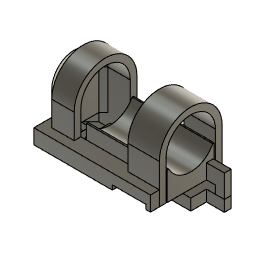
Laser Module Cover (Autodesk Fusion 360 design; units mm, degrees)
Autodesk Fusion 360 part; units mm, degrees
sketch "Sketch1" plane through (0, 0, 0) normal (1, 0, 0) x (0, 1, 0)
  line L0 (0, 0) -> (14, 0)
  line L1 (14, 0) -> (14, 8.8)
  line L2 (0, 0) -> (0, 8.8)
  arc A0 (14, 8.8) -> (0, 8.8) centre (7, 8.8) ccw
  dimension "d2" = 8.8
  dimension "d3" = 14
  constraint coincident L0.start L2.start
  constraint horizontal L0
  constraint perpendicular L0 L1
  constraint perpendicular L0 L2
  constraint tangent L1 A0
  constraint tangent L2 A0
  measures "d2" vertical distance of L0.start L2.end
  measures "d3" horizontal distance of L0.start L0.end
extrude "Extrude1" add sketch "Sketch1" along normal blind 1 makes body 1
sketch "Sketch2" plane through (1, 0, 0) normal (1, 0, 0) x (0, 1, 0)
  line L0 (0, 0) -> (14, 0)
  line L1 (14, 0) -> (14, 8.8)
  arc A0 (14, 8.8) -> (0, 8.8) centre (7, 8.8) ccw
  line L2 (0, 8.8) -> (0, 0)
  line L3 (1.5, 0) -> (1.5, 8.8)
  line L4 (12.5, 0) -> (12.5, 8.8)
  arc A1 (12.5, 8.8) -> (1.5, 8.8) centre (7, 8.8) ccw
  dimension "d6" = 1.5
  dimension "d7" = 1.5
  constraint coincident L0 L3.start
  constraint perpendicular L0 L3
  constraint coincident L0 L4.start
  constraint perpendicular L0 L4
  constraint coincident A0.centre A1.centre
  constraint tangent L3 A1
  measures "d6" distance of L2 L3
  measures "d7" distance of L1 L4
extrude "Extrude2" add sketch "Sketch2" along normal blind 6 contours L0 L1 A0 L2 L3 L4 A1 bodies 1
extrude "Extrude3" add 1 faces at (7, 13.5, 2.9333) along direction (1, 0, 0) blind 7 separate body on bodies 1 makes body 2
sketch "Sketch3" plane through (0, 0, 0) normal (0, 0, 1) x (1, 0, 0)
  line L0 (0, 0) -> (26, 0) construction
  dimension "d12" = 26
  constraint coincident L0.start origin
  measures "d12" distance of L0.start L0.end
move_body "Align1" bodies 2 to x (1, 0, 0) y (0, 1, 0) z (0, 0, 1) at (12, 0, 0)
sketch "Sketch4" plane through (0, 0, 0) normal (0, 0, -1) x (1, 0, 0)
  line L0 (0, 0) -> (0, -14)
  line L1 (0, -14) -> (7, -14)
  line L2 (7, -14) -> (7, -12.5)
  line L3 (7, -12.5) -> (1, -12.5)
  line L4 (1, -12.5) -> (1, -1.5)
  line L5 (1, -1.5) -> (7, -1.5)
  line L6 (7, -1.5) -> (7, 0)
  line L7 (7, 0) -> (0, 0)
  line L8 (0, -1.5) -> (26, -1.5)
  line L9 (26, -1.5) -> (26, 2)
  line L10 (26, 2) -> (0, 2)
  line L11 (0, 2) -> (0, -1.5)
  point P0 (26, -1.5)
  dimension "d13" = 3.5
  constraint coincident L0 L8.start
  constraint perpendicular L0 L8
  constraint perpendicular L8 L9
  constraint perpendicular L0 L10
  constraint perpendicular L8 L11
  constraint coincident P0 L8.end
  measures "d13" vertical distance of L8.start L10.end
extrude "Extrude4" add sketch "Sketch4" against normal blind 3.3 contours L6 L7 L8 L9 L10 L11 bodies 2 1
sketch "Sketch5" plane through (0, 0, 0) normal (0, 0, -1) x (1, 0, 0)
  line L0 (1, -1.5) -> (26, -1.5)
  line L1 (26, -1.5) -> (26, 0)
  line L2 (26, 0) -> (26, 2)
  line L3 (26, 2) -> (0, 2)
  line L4 (0, 2) -> (0, -14)
  line L5 (0, -14) -> (7, -14)
  line L6 (7, -14) -> (7, -12.5)
  line L7 (7, -12.5) -> (1, -12.5)
  line L8 (1, -12.5) -> (1, -1.5)
  line L9 (0, -14) -> (26, -14)
  line L10 (26, -14) -> (26, -12.5)
  line L11 (26, -12.5) -> (0, -12.5)
  line L12 (0, -12.5) -> (0, -14)
  point P0 (26, -12.5)
  constraint horizontal L9
  constraint vertical L10
  constraint horizontal L11
  constraint vertical L12
  constraint coincident P0 L10.end
  constraint coincident L4.end L5.start
extrude "Extrude5" add sketch "Sketch5" along normal blind 1.8 contours L4 L5 L6 L7 L9 L11 L12 | L6 L9 L10 L11 bodies 2
sketch "Sketch6" plane through (0, 0, 0) normal (0, 0, -1) x (1, 0, 0)
  line L0 (0, -12.5) -> (1, -12.5)
  line L1 (1, -12.5) -> (1, -1.5)
  line L2 (1, -1.5) -> (26, -1.5)
  line L3 (26, -1.5) -> (26, 0)
  line L4 (26, 0) -> (26, 2)
  line L5 (26, 2) -> (0, 2)
  line L6 (0, 2) -> (0, -12.5)
  line L7 (17.5, -1.5) -> (17.5, 2.5)
  line L8 (26, 2.5) -> (26, -1.5)
  line L9 (25, 2.5) -> (25, -1.5)
  line L10 (17.5, 2.5) -> (25, 2.5)
  line L11 (25, -1.5) -> (17.5, -1.5)
  dimension "d19" = 8.5
  dimension "d22" = 1
  constraint vertical L7
  constraint vertical L8
  constraint coincident L2 L9.end
  constraint horizontal L10
  constraint horizontal L11
  measures "d19" horizontal distance of L7.end L8.start
  measures "d22" distance of L8 L9
extrude "Extrude6" cut sketch "Sketch6" against normal blind 1 contours L5 L7 L9 L10 | L2 L5 L7 L9 L11 bodies 2
sketch "Sketch7" plane through (0, 0, -1.8) normal (0, 0, -1) x (1, 0, 0)
  line L0 (0, -12.5) -> (0, -14)
  line L1 (0, -14) -> (26, -14)
  line L2 (26, -14) -> (26, -12.5)
  line L3 (26, -12.5) -> (0, -12.5)
  line L4 (0, -14) -> (26, -14)
  line L5 (26, -14) -> (26, -7)
  line L6 (26, -7) -> (0, -7)
  line L7 (0, -7) -> (0, -14)
  line L8 (26, -14) -> (26, 0)
  dimension "d23" = 7
  constraint horizontal L4
  constraint vertical L5
  constraint horizontal L6
  constraint vertical L7
  constraint coincident L5.end L8
  constraint coincident L0.end L1.start
  measures "d23" vertical distance of L1.end L5.end
extrude "Extrude7" add sketch "Sketch7" along normal blind 2.5 bodies 2
sketch "Sketch8" plane through (0, 0, -1.8) normal (0, 0, 1) x (-1, 0, 0)
  line L0 (-26, -12.5) -> (0, -12.5)
  line L1 (0, -12.5) -> (0, -7)
  line L2 (0, -7) -> (-26, -7)
  line L3 (-26, -7) -> (-26, -12.5)
  line L4 (0, -12.5) -> (-2.5, -12.5)
  line L5 (-2.5, -12.5) -> (-2.5, -6)
  line L6 (-2.5, -6) -> (0, -6)
  line L7 (0, -6) -> (0, -12.5)
  dimension "d26" = 6.5
  dimension "d27" = 2.5
  constraint horizontal L4
  constraint vertical L5
  constraint horizontal L6
  constraint vertical L7
  constraint coincident L0.end L1.start
  measures "d26" vertical distance of L0.end L6.end
  measures "d27" distance of L0.end L4.end
extrude "Extrude8" cut sketch "Sketch8" against normal blind 1 contours L0 L1 L2 L4 L5 L7 | L2 L5 L6 L7 bodies 2
sketch "Sketch1 (2)" plane through (0, 0, 0) normal (1, 0, 0) x (0, 0, -1) in component "Laser Module Brace v2"
  line L0 (0, 0) -> (10.5, 0)
  line L1 (10.5, 0) -> (10.5, 3.3)
  line L2 (10.5, 3.3) -> (10.5, 6.3)
  line L3 (10.5, 3.3) -> (0, 3.3) construction
  line L4 (0, 0) -> (0, 6.3)
  line L5 (-1, 6.3) -> (11.5, 6.3) construction
  line L6 (0, 6.3) -> (0.3715, 6.3)
  line L7 (10.1985, 6.3) -> (10.5, 6.3)
  arc A0 (0.3715, 6.3) -> (5.285, 3.3) centre (5.285, 8.8237) ccw
  arc A1 (5.285, 3.3) -> (10.1985, 6.3) centre (5.285, 8.8237) ccw
  arc A2 (10.785, 8.8237) -> (-0.215, 8.8237) centre (5.285, 8.8237) ccw
  dimension "d1" = 10.5
  dimension "d17_1" = 3
  dimension "d18" = 3.3
  constraint coincident L0.start L4.start
  constraint perpendicular L2 L3
  constraint perpendicular L0 L4
  constraint tangent L3 A0
  constraint perpendicular L2 L5
  constraint coincident L5 L4.end
  constraint coincident L5 L6.end
  constraint perpendicular L4 L6
  constraint coincident L5 L7.start
  constraint coincident L7.start A0
  constraint coincident L5 L2.end
  constraint coincident L3 A0.end
  constraint concentric A0 A1
  constraint concentric A0 A2
  constraint collinear L1 L2
  constraint horizontal L0
  measures "d1" distance of L0.start L0.end
  measures "d17_1" distance of L3 L5
  measures "d18" distance of L0.start L3
extrude "Extrude1'" add sketch "Sketch1 (2)" along normal blind 18 separate body makes body 3 in component "Laser Module Brace v2"
sketch "Sketch2 (2)" plane through (0, 0, 0) normal (0, -1, 0) x (1, 0, 0) in component "Laser Module Brace v2"
  line L0 (0, 0) -> (0, -10.5)
  line L1 (0, -10.5) -> (18, -10.5)
  line L2 (18, -10.5) -> (18, 0)
  line L3 (18, 0) -> (0, 0)
  circle A0 centre (4.52, -8.9566) radius 0.8
  circle A1 centre (14.52, -8.9566) radius 0.8
  circle A2 centre (4.52, -6.04) radius 0.8
  circle A3 centre (14.52, -6.04) radius 0.8
  point P0 (0, -10.5)
  dimension "d7_1" = 1.6
  dimension "d8_1" = 1.6
  dimension "d9_1" = 1.6
  dimension "d10_1" = 1.6
  dimension "d11_1" = 4.52
  dimension "d12_1" = 14.52
  dimension "d13_1" = 1.5433
  dimension "d14_1" = 4.46
  constraint coincident P0 L0.end
  constraint vertical A0.centre A2.centre
  constraint vertical A1.centre A3.centre
  constraint horizontal A2.centre A3.centre
  constraint horizontal A0.centre A1.centre
  measures "d7_1" diameter of A0
  measures "d8_1" diameter of A1
  measures "d9_1" diameter of A2
  measures "d10_1" diameter of A3
  measures "d11_1" horizontal distance of P0 A0.centre
  measures "d12_1" horizontal distance of P0 A1.centre
  measures "d13_1" vertical distance of P0 A0.centre
  measures "d14_1" vertical distance of P0 A2.centre
extrude "Extrude2'" add sketch "Sketch2 (2)" along normal blind 1.6 contours A0 | A1 | A2 | A3 bodies 3 in component "Laser Module Brace v2"
sketch "Sketch3 (2)" plane through (0, 0, 0) normal (1, 0, 0) x (0, 0, -1) in component "Laser Module Brace v2"
copy_body "Body->Comp1" bodies 2 removing the originals makes body 4 in component "Laser Module Frame"
sketch "Sketch9" plane through (0, 0, -1.8) normal (0, 0, 1) x (-1, 0, 0)
  line L0 (0, -7) -> (-2.5, -7)
  line L1 (-2.5, -7) -> (-2.5, -12.5)
  line L2 (-2.5, -12.5) -> (0, -12.5)
  line L3 (0, -12.5) -> (0, -7)
  line L4 (0, -14) -> (4, -14)
  line L5 (4, -14) -> (4, -10.5)
  line L6 (4, -10.5) -> (0, -10.5)
  line L7 (0, -10.5) -> (0, -14)
  line L8 (0, -12.5) -> (-2.5, -12.5)
  line L9 (0, -12.5) -> (2, -10.5)
  line L10 (-13, -18.3426) -> (-13, 22.3426) construction
  line L11 (0, 2) -> (-26, 2)
  line L12 (-26, -14) -> (-30, -14)
  line L13 (-30, -14) -> (-30, -10.5)
  line L14 (-30, -10.5) -> (-26, -10.5)
  line L15 (-26, -12.5) -> (-28, -10.5)
  line L16 (-26, -10.5) -> (-26, -14)
  line L17 (-2.5, -12.5) -> (-2.5, -7)
  line L18 (-2.5, -7) -> (-26, -7)
  line L19 (-26, -7) -> (-26, -12.5)
  line L20 (-26, -12.5) -> (-2.5, -12.5)
  point P0 (0, -14)
  dimension "d33" = 4
  dimension "d34" = 3.5
  dimension "d35" = 45
  constraint horizontal L4
  constraint vertical L5
  constraint horizontal L6
  constraint vertical L7
  constraint coincident P0 L4.start
  constraint coincident L2.end L3.start
  constraint coincident L6 L9.end
  constraint vertical L10
  constraint midpoint L10 L11
  constraint symmetric P0 L10 L12.start
  constraint symmetric L4.end L10 L12.end
  constraint symmetric L5.end L10 L13.end
  constraint symmetric L6.end L10 L14.end
  constraint symmetric L2.end L10 L15.start
  constraint symmetric L9.end L10 L15.end
  measures "d33" distance of P0 L4.end
  measures "d34" distance of L4.end L5.end
  measures "d35" angle of L7 L9
extrude "Extrude1''" add sketch "Sketch9" against normal up to surface (2.5 mm away) contours L3 L6 L7 L9 | L4 L5 L6 L7 L9 | L12 L13 L14 L15 L16 | L14 L15 L16 L19 bodies 4 in component "Laser Module Frame"
extrude "Extrude3'" add sketch "Sketch9" along normal up to surface (5.1 mm away) contours L12 L13 L14 L15 L16 | L14 L15 L16 L19 sketch seen with x (1, 0, 0) y (0, 0, -1) z (0, 1, 0) at (-8, 0.0237, 1.715) bodies 3 in component "Laser Module Brace v2"
extrude "Extrude4'" cut sketch "Sketch9" along normal up to surface (1.7763 mm away) contours L14 L15 L16 L19 sketch seen with x (1, 0, 0) y (0, 0, -1) z (0, 1, 0) at (-8, 0.0237, 1.715) bodies 3 in component "Laser Module Brace v2"
extrude "Extrude2''" add sketch "Sketch9" along normal up to surface (5.1 mm away) contours L3 L6 L7 L9 | L4 L5 L6 L7 L9 bodies 4 in component "Laser Module Frame"
extrude "Extrude3''" cut sketch "Sketch9" along normal up to surface (1.8 mm away) and the other way up to surface (1 mm away) contours L3 L6 L7 L9 bodies 4 in component "Laser Module Frame"
chamfer "Chamfer1" distance 2 angle 45 7 edges at (-4, 14, -0.5) (13, 14, -4.3) (30, 14, -3.05) (-2, 14, 3.3) (0, 14, 6.05) (0, 7, 15.8) (0, 0, 6.05) on bodies 4 in component "Laser Module Frame"
chamfer "Chamfer1'" distance 2 angle 45 2 edges at (22, 0.7737, -12.285) (20, 3.3237, -12.285) on bodies 3 in component "Laser Module Brace v2"
chamfer "Chamfer2" distance 1 angle 45 3 edges at (1, 12.5, 4.4) (1, 7, 14.3) (1, 1.5, 4.4) on bodies 4 in component "Laser Module Frame"
component "Laser Module Brace v2" placed x (1, 0, 0) y (0, 0, 1) z (0, -1, 0) at (8, 1.715, -0.0237)
component "Laser Module Frame" placed x (1, 0, 0) y (0, 1, 0) z (0, 0, 1) at (0, 0, 0)
equation "d2 = 6.5 mm + 2.3 mm"
equation "d34 = 2 mm + 1.5 mm"
